Ofenstoepsel_v1 (Autodesk Fusion 360 design; units mm, degrees)
Autodesk Fusion 360 part; units mm, degrees
sketch "Sketch1" plane through (0, 0, 0) normal (0, 1, 0) x (1, 0, 0)
  circle A0 centre (0, 0) radius 3.1
  circle A1 centre (0, 0) radius 18
  line L0 (-20, 0) -> (-20, 15)
  line L1 (-20, 15) -> (20, 15)
  line L2 (-3.1, 0) -> (-3.1, 26.7425)
  line L3 (3.1, 0) -> (3.1, 30)
  dimension "d1" = 6.2
  dimension "d2" = 36
  dimension "d3" = 15
  constraint coincident A0.centre A1.centre
  constraint vertical L0
  constraint perpendicular L0 L1
  constraint coincident A0 L2.start
  constraint tangent A0 L2
  constraint perpendicular L1 L2
  constraint coincident A0 L3.start
  constraint tangent A0 L3
  constraint perpendicular L1 L3
  measures "d1" diameter of A0
  measures "d2" diameter of A1
  measures "d3" distance of L0.start L0.end
extrude "Extrude1" add sketch "Sketch1" along normal blind 29 contours A0 A1 L1 L2 L3 | A0 L1 L2 L3 | A1 L1 L3 | A1 L1 L2 L3 | A1 L1 L2 makes body 1
extrude "Extrude2" add sketch "Sketch1" against normal blind 5 separate body contours A0 A1 L1 L2 L3 | A0 L1 L2 L3 makes body 2
ref_plane "WorkPlane1" through (0, -15, 0) normal (0, 1, 0) x (1, 0, 0)
sketch "Sketch2" plane through (0, -15, 0) normal (0, 1, 0) x (1, 0, 0)
  circle A0 centre (0, 0) radius 18
  line L0 (-20, 15) -> (20, 15)
  line L1 (3.1, 0) -> (3.1, 30)
  line L2 (-3.1, 0) -> (-3.1, 26.7425)
  circle A1 centre (0, 0) radius 3.1
extrude "Extrude3" add sketch "Sketch2" along normal blind 10 separate body contours A0 L0 L1 L2 A1 makes body 3
extrude "Extrude4" add 1 faces at (-7.9758, 29, -10.2666) along direction (0, 1, 0) blind 8 on bodies 1 bodies 1
fillet "Fillet1" radius 12 1 edges at (-16.7819, 37, 6.5091) on bodies 1
